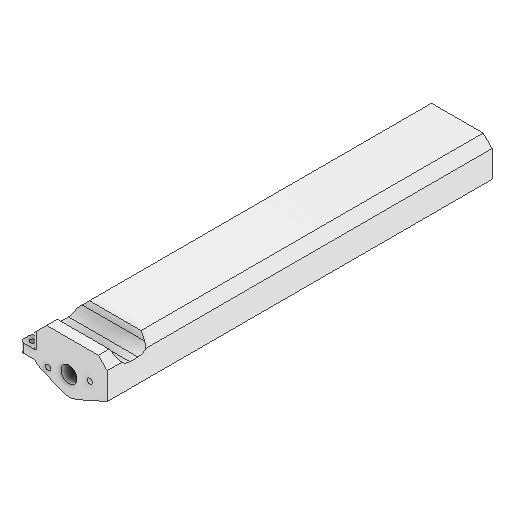
# Autodesk Inventor part: LeadScrewArch
Saved by Autodesk Inventor 2026.2 (Build 302298000, 298)
## iProperties
Created: 2026-03-31
Part Number: LeadScrewArch
Material: ABS Plastic
Document SubType Name: Modeling
Designer: gaoet
Density: 1.06 g/cm^3
Appearance: Smooth - White
Author: gaoet
Autodesk Inventor part; units mm, degrees
ref_plane "YZ Plane" through (0, 0, 0) normal (1, 0, 0) x (0, 1, 0)
ref_plane "XZ Plane" through (0, 0, 0) normal (0, 1, 0) x (-1, 0, 0)
ref_plane "XY Plane" through (0, 0, 0) normal (0, 0, 1) x (1, 0, 0)
sketch "Sketch1" plane through (0, 0, 0) normal (0, 0, 1) x (1, 0, 0)
  line L0 (-21.5, -10) -> (21.5, -10)
  line L1 (21.5, -10) -> (21.5, 10)
  line L2 (21.5, 10) -> (-21.5, 10)
  line L3 (-21.5, 10) -> (-21.5, -10)
  line L4 (-21.5, -10) -> (21.5, 10) construction
  line L5 (21.5, -10) -> (-21.5, 10) construction
  circle A0 centre (0, -7.5) radius 13.25
  line L6 (-13.25, -7.5) -> (-13.25, -10)
  line L7 (13.25, -7.5) -> (13.25, -10)
  point P0 (0, 0)
  point P1 (0, 10)
  dimension "d0" = 21.5
  dimension "d1" = 2.5
  dimension "d2" = 26.5
  dimension "d3" = 10
  constraints: 16 end point, 3 midpoint, 2 parallel, 2 point on circle, 2 point on line, 2 tangent, 2 vertical, 1 centre point, 1 horizontal, 1 perpendicular, 1 vertical alignment
  measures "d0" distance from line of L3 point (0, 0)
  measures "d1" distance from line of L0 A0.centre
  measures "d2" diameter of A0
  measures "d3" distance of point (0, 10) point (0, 0)
extrude "Extrusion1" add sketch "Sketch1" along normal blind 200 contours L3 L2 L1 L0 L7 A0 L6
sketch "Sketch2" plane through (13.25, -10, 0) normal (0, -1, 0) x (1, 0, 0)
  line L0 (-34.75, 0) -> (-34.75, 200) projected
  line L1 (-26.5, 0) -> (-26.5, 200) projected
  line L2 (-34.75, 100) -> (-26.5, 100)
  line L3 (8.25, 0) -> (8.25, 200) projected
  point P0 (-13.25, 0)
  point P1 (-30.625, 180)
  point P2 (4.125, 180)
  point P3 (-30.625, 60)
  point P4 (4.125, 60)
  point P5 (-30.625, 140)
  point P6 (4.125, 140)
  point P7 (-30.625, 100)
  point P8 (4.125, 100)
  point P9 (-30.625, 20)
  point P10 (4.125, 20)
  dimension "d6" = 8.25
  dimension "d7" = 4.125
  dimension "d8" = 200
  dimension "d9" = 20
  dimension "d10" = 40
  dimension "d11" = 40
  dimension "d12" = 40
  dimension "d13" = 4.125
  dimension "d14" = 40
  constraints: 10 vertical alignment, 5 horizontal alignment, 2 end point, 2 midpoint
  measures "d6" distance between parallel lines of L0 L1
  measures "d7" distance from line of L0 point (-30.625, 180)
  measures "d8" distance of L0.start L0.end
  measures "d9" vertical distance of L0.end point (-30.625, 180)
  measures "d10" distance of point (-30.625, 180) point (-30.625, 140)
  measures "d11" distance of point (-30.625, 100) point (-30.625, 140)
  measures "d12" distance of point (-30.625, 60) point (-30.625, 100)
  measures "d13" distance from line of L3 point (4.125, 180)
  measures "d14" distance of point (-30.625, 20) point (-30.625, 60)
hole "Hole1" at (17.375, -10, 180) at (17.375, -10, 60) at (17.375, -10, 140) at (17.375, -10, 100) at (17.375, -10, 20) direction (0, 1, 0) diameter 4 depth 12
sketch "Sketch3" plane through (0, 0, 200) normal (0, 0, 1) x (1, 0, 0)
  line L0 (21.5, 10) -> (-21.5, 10) projected
  line L1 (-21.5, 10) -> (-21.5, -10) projected
  line L2 (-21.5, -10) -> (-13.25, -10) projected
  line L3 (-13.25, -10) -> (-13.25, -7.5) projected
  arc A0 (13.25, -7.5) -> (-13.25, -7.5) centre (0, -7.5) ccw projected
  line L4 (13.25, -7.5) -> (13.25, -10) projected
  line L5 (13.25, -10) -> (21.5, -10) projected
  line L6 (21.5, -10) -> (21.5, 10) projected
  circle A1 centre (0, -7.5) radius 8
  circle A2 centre (0, -7.5) radius 11
  line L7 (21.5, -10) -> (4.4586, -17.5559)
  line L8 (-21.5, -10) -> (-4.4586, -17.5559)
  circle A3 centre (0, -7.5) radius 4.5
  point P0 (0, 0)
  dimension "d23" = 16
  dimension "d24" = 3
  dimension "d25" = 9
  constraints: 4 end point, 3 centre point, 3 coincident, 2 point on circle, 2 tangent
  measures "d23" diameter of A1
  measures "d24" radial gap between concentric circles of A2 A1
  measures "d25" diameter of A3
extrude "Extrusion2" add sketch "Sketch3" against normal blind 8 contours L7 A2 L8 L2 L3 A0 L4 L5 | A2 | A1
sketch "Sketch4" plane through (0, 0, 192) normal (0, 0, -1) x (-1, 0, 0)
  line L0 (-21.5, -10) -> (-4.4586, -17.5559) projected
  arc A0 (-4.4586, -17.5559) -> (4.4586, -17.5559) centre (0, -7.5) ccw projected
  line L1 (4.4586, -17.5559) -> (21.5, -10) projected
  line L2 (13.25, -10) -> (21.5, -10) projected
  line L3 (13.25, -7.5) -> (13.25, -10) projected
  arc A1 (13.25, -7.5) -> (-13.25, -7.5) centre (0, -7.5) ccw projected
  line L4 (-13.25, -10) -> (-13.25, -7.5) projected
  line L5 (-21.5, -10) -> (-13.25, -10) projected
  circle A2 centre (0, -7.5) radius 4.5 projected
  circle A3 centre (0, -7.5) radius 8
  point P0 (0, 0)
  dimension "d28" = 16
  constraints: 1 centre point, 1 coincident
  measures "d28" diameter of A3
extrude "Extrusion3" cut sketch "Sketch4" against normal blind 5 contours A3
sketch "Sketch5" plane through (0, -7.5, 197) normal (0, 0, -1) x (-1, 0, 0)
  circle A0 centre (0, 0) radius 8 projected
  circle A1 centre (0, 0) radius 4.5 projected
  circle A2 centre (0, 0) radius 6.5
  point P0 (0, 7.5)
  dimension "d31" = 1.5
  constraints: 1 centre point
  measures "d31" radial gap between concentric circles of A0 A2
extrude "Extrusion4" cut sketch "Sketch5" against normal blind 0.75 contours A2
chamfer "Chamfer1" distance 5 angle 45 1 edges at (21.5, 10, 100)
sketch "Sketch6" plane through (-21.5, -10, 0) normal (-1, 0, 0) x (0, 0, 1)
  line L0 (0, 30.7296) -> (208.3167, 30.7296)
  line L1 (208.3167, 30.7296) -> (208.3167, -9.5773)
  line L2 (208.3167, -9.5773) -> (0, -9.5773)
  line L3 (0, -9.5773) -> (0, 30.7296)
  point P0 (0, 10)
  constraints: 8 end point, 2 parallel, 1 horizontal, 1 perpendicular
extrude "Extrusion5" cut sketch "Sketch6" against normal blind 4
chamfer "Chamfer2" distance 5 angle 45 1 edges at (-17.5, 10, 100)
sketch "Sketch7" plane through (-13.25, -10, 0) normal (0, -1, 0) x (1, 0, 0)
  line L0 (-4.25, 192) -> (-4.25, 0) projected
  line L1 (-4.25, 0) -> (0, 0) projected
  line L2 (0, 0) -> (0, 192) projected
  line L3 (0, 192) -> (-4.25, 192) projected
  point P0 (13.25, 0)
extrude "Extrusion6" add sketch "Sketch7" along normal blind 11
sketch "Sketch8" plane through (-17.5, -10, 0) normal (-1, 0, 0) x (0, 0, 1)
  line L0 (0, 15) -> (200, 15) projected
  line L1 (0, -11) -> (0, 15) projected
  line L2 (192, -11) -> (0, -11) projected
  line L3 (192, -1.7735) -> (192, -11) projected
  line L4 (200, -1.7735) -> (192, -1.7735) projected
  line L5 (200, 15) -> (200, -1.7735) projected
  line L6 (192, -11) -> (0, -11)
  line L7 (0, -11) -> (0, 0)
  line L8 (0, 0) -> (192, 0)
  line L9 (192, 0) -> (192, -11)
  point P0 (0, 10)
  dimension "d45" = 11
  constraints: 8 end point, 2 parallel, 1 horizontal, 1 perpendicular, 1 point on line
  measures "d45" distance between parallel lines of L2 L8
extrude "Extrusion7" add sketch "Sketch8" along normal blind 2.75 contours L8 L9 L3 L2 L1
chamfer "Chamfer3" distance 2.75 angle 45 1 edges at (-20.25, -10, 96)
sketch "Sketch9" plane through (-13.25, -7.5, 192) normal (1, 0, 0) x (0, 0, -1)
  line L0 (0, -6.1579) -> (0, 0) projected
  line L1 (0, -6.1579) -> (0, -13.5) projected
  line L2 (192, -13.5) -> (0, -13.5) projected
  line L3 (192, 0) -> (192, -13.5) projected
  line L4 (192, 0) -> (0, 0) projected
  line L5 (174, -2.5) -> (170, -2.5) projected
  line L6 (170, 9.5) -> (174, 9.5) projected
  point P0 (192, 7.5)
  point P1 (172, -8.5)
  point P2 (132, -8.5)
  point P3 (92, -8.5)
  point P4 (52, -8.5)
  point P5 (12, -8.5)
  dimension "d51" = 13.5
  dimension "d52" = 5
  dimension "d53" = 20
  dimension "d56" = 40
  constraints: 1 horizontal, 4 other
  measures "d51" distance between parallel lines of L2 L4
  measures "d52" distance from line of L2 point (172, -8.5)
  measures "d53" distance from line of L3 point (172, -8.5)
  measures "d56" distance of point (172, -8.5) point (132, -8.5)
hole "Hole2" at (-13.25, -16, 20) at (-13.25, -16, 60) at (-13.25, -16, 100) at (-13.25, -16, 140) at (-13.25, -16, 180) direction (-1, 0, 0) diameter 3 depth 12 counterbore diameter 5.75 counterbore depth 3
sketch "Sketch10" plane through (0, 0, 200) normal (0, 0, 1) x (1, 0, 0)
  line L0 (-17.5, 5) -> (-12.5, 10) projected
  line L1 (-17.5, 5) -> (-17.5, -11.7735) projected
  line L2 (-17.5, -11.7735) -> (-4.4586, -17.5559) projected
  arc A0 (-4.4586, -17.5559) -> (4.4586, -17.5559) centre (0, -7.5) ccw projected
  line L3 (4.4586, -17.5559) -> (21.5, -10) projected
  line L4 (21.5, -10) -> (21.5, 5) projected
  line L5 (16.5, 10) -> (21.5, 5) projected
  line L6 (16.5, 10) -> (-12.5, 10) projected
  circle A1 centre (0, -7.5) radius 4.5 projected
  point P0 (0, 0)
extrude "Extrusion8" add sketch "Sketch10" along normal blind 16
sketch "Sketch11" plane through (0, 0, 216) normal (0, 0, 1) x (1, 0, 0)
  arc A0 (-4.4586, -17.5559) -> (4.4586, -17.5559) centre (0, -7.5) ccw projected
  line L0 (4.4586, -17.5559) -> (21.5, -10) projected
  line L1 (21.5, -10) -> (21.5, 5) projected
  line L2 (21.5, 5) -> (16.5, 10) projected
  line L3 (16.5, 10) -> (-12.5, 10) projected
  line L4 (-12.5, 10) -> (-17.5, 5) projected
  line L5 (-17.5, 5) -> (-17.5, -11.7735) projected
  line L6 (-17.5, -11.7735) -> (-4.4586, -17.5559) projected
  circle A1 centre (0, -7.5) radius 4.5 projected
  line L7 (0, -7.5) -> (0, 10)
  line L8 (-11.7378, -9.9949) -> (0, -7.5)
  line L9 (11.7378, -5.0051) -> (0, -7.5)
  dimension "d80" = 12
  dimension "d81" = 102
  constraints: 6 end point, 2 collinear, 1 point on line, 1 vertical
  measures "d80" distance of L8.start L7.start
  measures "d81" angle of L7 L8
hole "Hole3" at (-11.7378, -9.9949, 216) at (11.7378, -5.0051, 216) direction (0, 0, -1) diameter 3 depth 15
sketch "Sketch13" plane through (-17.5, -10, 0) normal (-1, 0, 0) x (0, 0, 1)
  line L0 (0, 0) -> (192, 0) projected
  line L1 (192, 0) -> (192, -1.7735) projected
  line L2 (216, -1.7735) -> (192, -1.7735) projected
  line L3 (216, 15) -> (216, -1.7735) projected
  line L4 (0, 15) -> (216, 15) projected
  line L5 (0, 0) -> (0, 15) projected
  line L6 (216, 5) -> (209, 5)
  line L7 (209, 5) -> (209, 0)
  line L8 (209, 0) -> (216, 0)
  line L9 (216, 0) -> (216, 5)
  line L10 (216, 15) -> (216, -1.7735) projected
  line L11 (216, 20) -> (0, 20) projected
  point P0 (0, 10)
  point P1 (212.5, 0)
  point P2 (216, 0)
  dimension "d82" = 20
  dimension "d83" = 7
  dimension "d84" = 5
  constraints: 8 end point, 2 parallel, 1 collinear, 1 horizontal, 1 midpoint, 1 perpendicular
  measures "d82" distance from line of L11 point (212.5, 0)
  measures "d83" distance of L6.start L6.end
  measures "d84" distance of L6.end L7.end
extrude "Extrusion9" add sketch "Sketch13" along normal blind 10 contours L3 L8 L7 L6
chamfer "Chamfer4" distance 1.7735 angle 45 1 edges at (-17.5, -10, 212.5)
chamfer "Chamfer5" distance 10 angle 45 1 edges at (-17.5, -5, 212.5)
sketch "Sketch14" plane through (-12.5, 10, 0) normal (0, 1, 0) x (1, 0, 0)
  line L0 (0, -216) -> (0, 0) projected
  line L1 (0, 0) -> (-5, 0) projected
  line L2 (-5, 0) -> (-5, -209) projected
  line L3 (-5, -209) -> (-15, -209) projected
  line L4 (-15, -216) -> (-15, -209) projected
  line L5 (0, -216) -> (-15, -216) projected
  point P0 (12.5, 0)
  point P1 (-11.375, -212.5)
  dimension "d93" = 7
  dimension "d94" = 3.5
  dimension "d95" = 3.625
  measures "d93" distance of L4.start L3.end
  measures "d94" distance from line of L5 point (-11.375, -212.5)
  measures "d95" distance from line of point (-11.375, -212.5) L4
hole "Hole4" at (-23.875, 10, 212.5) direction (0, -1, 0) diameter 3 depth 30 counterbore diameter 7.25 counterbore depth 15
sketch "Sketch15" plane through (-24.8187, -5, 209) normal (0, 1, 0) x (1, 0, 0)
  circle A0 centre (0.9437, -3.5) radius 1.5 projected
  line L0 (0, 0) -> (1.8875, 0) projected
  arc A1 (0, 0) -> (-2.6813, -3.5) centre (0.9437, -3.5) ccw projected
  arc A2 (-2.6813, -3.5) -> (0, -7) centre (0.9437, -3.5) ccw projected
  line L1 (1.8875, -7) -> (0, -7) projected
  arc A3 (1.8875, -7) -> (1.8875, 0) centre (0.9437, -3.5) ccw projected
  arc A4 (-2.6813, -3.5) -> (0, -7) centre (0.9437, -3.5) ccw projected
  line L2 (-2.6813, -7) -> (-2.6813, -3.5) projected
  line L3 (0, -7) -> (-2.6813, -7) projected
  arc A5 (0, 0) -> (-2.6813, -3.5) centre (0.9437, -3.5) ccw projected
  line L4 (0, 0) -> (-2.6813, 0) projected
  line L5 (-2.6813, -3.5) -> (-2.6813, 0) projected
  point P0 (24.8187, 209)
  point P1 (-2.6813, -3.5)
  point P2 (-2.6813, -3.5)
  point P3 (-2.6813, -3.5)
  point P4 (-2.6813, -3.5)
  point P5 (-2.6813, -3.5)
extrude "Extrusion10" cut sketch "Sketch15" along normal blind 9.25 contours A1 L5 L4 | A2 L3 L2
fillet "Fillet3" radius 2 4 edges at (-22.9313, -2.7157, 209) (-22.9313, -2.7157, 216) (-27.5, -7.5, 209) (-27.5, -7.5, 216)
sketch "Sketch16" plane through (-17.5, -10, 0) normal (-1, 0, 0) x (0, 0, 1)
  line L0 (192, 10.5) -> (197, 10.5) projected
  line L1 (197.75, 7) -> (216, 7) projected
  line L2 (216, 20) -> (0, 20) projected
  line L3 (192, 20) -> (194.481, 13)
  line L4 (194.481, 13) -> (207.519, 13)
  line L5 (207.519, 13) -> (210, 20)
  point P0 (0, 10)
  dimension "d106" = 7
  dimension "d107" = 18
  dimension "d108" = 6
  constraints: 6 end point, 2 point on line, 1 equal length, 1 parallel
  measures "d106" distance between parallel lines of L2 L4
  measures "d107" distance of L5.end L3.start
  measures "d108" distance of L2.start L5.end
extrude "Extrusion11" cut sketch "Sketch16" against normal through all
fillet "Fillet4" radius 6 2 edges at (2, 3, 194.481) (2, 3, 207.519)
equation "\"d7\" = 0.5 * d6"
equation "\"d9\" = 0.1 * d8"
equation "\"d10\" = 2 * d9"
equation "\"d11\" = d10"
equation "\"d12\" = d11"
equation "\"d13\" = d7"
equation "\"d14\" = d12"
equation "\"d94\" = 0.5 * d93"
body "Solid1"
